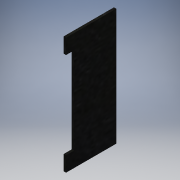
# Autodesk Inventor part: upper insert
Saved by Autodesk Inventor 2019 (Build 230136000, 136)
## iProperties
Created: 2020-03-06
Part Number: upper insert
Material: Generic
Document SubType Name: Modeling
Designer: ntb11189
Density: 1 g/cm^3
Appearance: Smooth - Black
Author: ntb11189
Autodesk Inventor part; units mm, degrees
ref_plane "YZ Plane" through (0, 0, 0) normal (1, 0, 0) x (0, 1, 0)
ref_plane "XZ Plane" through (0, 0, 0) normal (0, 1, 0) x (-1, 0, 0)
ref_plane "XY Plane" through (0, 0, 0) normal (0, 0, 1) x (1, 0, 0)
sketch "Sketch1" plane through (0, 0, 0) normal (1, 0, 0) x (0, 1, 0)
  line L0 (0, 0) -> (-116.5, 0)
  line L1 (-116.5, 0) -> (-116.5, -50)
  line L2 (-116.5, -50) -> (0, -50)
  line L3 (0, -50) -> (0, 0)
  line L4 (-15, 0) -> (-101.5, 0)
  line L5 (-101.5, 0) -> (-101.5, -8)
  line L6 (-101.5, -8) -> (-15, -8)
  line L7 (-15, -8) -> (-15, 0)
  dimension "d0" = 116.5
  dimension "d1" = 50
  dimension "d4" = 8
  dimension "d5" = 15
  dimension "d6" = 15
  constraints: 16 end point, 4 parallel, 2 horizontal, 2 perpendicular, 1 point on line
  measures "d0" distance of L2.end L1.end
  measures "d1" distance of L0.end L1.end
  measures "d4" distance of L5.end L4.end
  measures "d5" distance between parallel lines of L3 L7
  measures "d6" distance between parallel lines of L1 L5
extrude "Extrusion2" add sketch "Sketch1" along normal blind 2.3 contours L3 L2 L1 L0 L5 L6 L7
body "Solid2"
